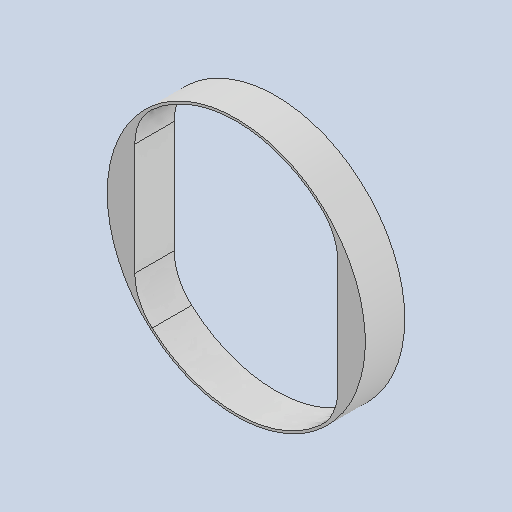
# Autodesk Inventor part: encoderring
Saved by Autodesk Inventor 2022 (Build 260153000, 153)
## iProperties
Created: 2022-03-19
Part Number: encoderring
Material: Generic
Document SubType Name: Modeling
Designer: zac-h
Density: 1 g/cm^3
Appearance: Default
Author: zac-h
Autodesk Inventor part; units mm, degrees
ref_plane "YZ Plane" through (0, 0, 0) normal (1, 0, 0) x (0, 1, 0)
ref_plane "XZ Plane" through (0, 0, 0) normal (0, 1, 0) x (-1, 0, 0)
sketch "Sketch1" plane through (0, 0, 0) normal (0, 0, 1) x (1, 0, 0)
  arc A0 (8.9281, 30.3907) -> (-8.9281, 30.3907) centre (0, 23.7533) ccw projected
  arc A1 (21.0435, 23.6744) -> (8.9281, 30.3907) centre (0, 0) ccw projected
  arc A2 (25.3062, 14.1822) -> (21.0435, 23.6744) centre (12.6062, 14.1822) ccw projected
  line L0 (25.3062, 14.1822) -> (25.3062, -14.1822) projected
  arc A3 (21.0435, -23.6744) -> (25.3062, -14.1822) centre (12.6062, -14.1822) ccw construction
  arc A4 (8.9281, -30.3907) -> (21.0435, -23.6744) centre (0, 0) ccw projected
  arc A5 (-8.9281, -30.3907) -> (8.9281, -30.3907) centre (0, -23.7533) ccw projected
  arc A6 (-21.0435, -23.6744) -> (-8.9281, -30.3907) centre (0, 0) ccw projected
  arc A7 (-25.3062, -14.1822) -> (-21.0435, -23.6744) centre (-12.6062, -14.1822) ccw projected
  line L1 (-25.3062, -14.1822) -> (-25.3062, 14.1822) projected
  arc A8 (-21.0435, 23.6744) -> (-25.3062, 14.1822) centre (-12.6062, 14.1822) ccw projected
  arc A9 (-8.9281, 30.3907) -> (-21.0435, 23.6744) centre (0, 0) ccw projected
  circle A10 centre (0, 0) radius 35.025 projected
  circle A11 centre (0, 0) radius 31.675 construction
  line L2 (25.7062, -14.1822) -> (25.7062, 14.1822)
  arc A12 (25.7062, 14.1822) -> (21.3093, 23.9733) centre (12.6062, 14.1822) ccw
  arc A13 (21.3093, 23.9733) -> (9.1683, 30.7368) centre (0, 0) ccw
  arc A14 (9.1683, 30.7368) -> (-9.1683, 30.7368) centre (0, 23.7533) ccw construction
  arc A15 (-9.1683, 30.7368) -> (-21.3093, 23.9733) centre (0, 0) ccw
  arc A16 (-21.3093, 23.9733) -> (-25.7062, 14.1822) centre (-12.6062, 14.1822) ccw
  line L3 (-25.7062, 14.1822) -> (-25.7062, -14.1822)
  arc A17 (-25.7062, -14.1822) -> (-21.3093, -23.9733) centre (-12.6062, -14.1822) ccw
  arc A18 (-21.3093, -23.9733) -> (-9.1683, -30.7368) centre (0, 0) ccw
  arc A19 (-9.1683, -30.7368) -> (9.1683, -30.7368) centre (0, -23.7533) ccw construction
  arc A20 (9.1683, -30.7368) -> (21.3093, -23.9733) centre (0, 0) ccw
  arc A21 (21.3093, -23.9733) -> (25.7062, -14.1822) centre (12.6062, -14.1822) ccw
  circle A22 centre (0, 0) radius 32.675
  circle A23 centre (0, 0) radius 32.075
  point P0 (-9.1683, -30.7368)
  point P1 (-9.1683, 30.7368)
  point P2 (9.1683, 30.7368)
  dimension "d20" = 0.4
  dimension "d21" = 1
  constraints: 20 point on circle, 11 centre point, 4 end point, 2 coincident, 17 other
  measures "d20" distance between parallel lines of L0 L2
ref_plane "Work Plane1" through (-72.8034, -89.1781, 10) normal (0, 0, 1) x (0.7418, 0.6706, 0)
extrude "Extrusion1" add sketch "Sketch1" along normal up to surface (10 mm away) contours A23 A0 A22 | A0 A22 A5 A23 A20 A13 | A23 A15 A18 A5 A22 A0 | A23 A21 L2 A12 | A5 A23 A22 | A16 L3 A17 A23
body "Solid1"
